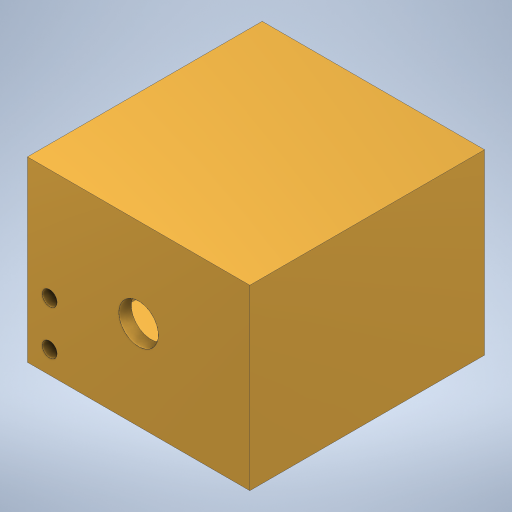
# Autodesk Inventor part: HUDISN-1-53
Saved by Autodesk Inventor 2024.2 (Build 282272000, 272)
## iProperties
Created: 2024-10-24
Part Number: HUDISN-1-53
Material: Generic
Document SubType Name: Modeling
Designer: Precisión-05
Density: 1 g/cm^3
Appearance: Default
Author: Precisión-05
Autodesk Inventor part; units mm, degrees
ref_plane "YZ Plane" through (0, 0, 0) normal (1, 0, 0) x (0, 1, 0)
ref_plane "XZ Plane" through (0, 0, 0) normal (0, 1, 0) x (-1, 0, 0)
ref_plane "XY Plane" through (0, 0, 0) normal (0, 0, 1) x (1, 0, 0)
sketch "Sketch1" plane through (0, 0, 0) normal (0, 1, 0) x (-1, 0, 0)
  line L0 (-22.5, 18) -> (22.5, 18)
  line L1 (22.5, 18) -> (22.5, -18)
  line L2 (22.5, -18) -> (-22.5, -18)
  line L3 (-22.5, -18) -> (-22.5, 18)
  line L4 (-22.5, 18) -> (22.5, -18) construction
  line L5 (22.5, 18) -> (-22.5, -18) construction
  line L6 (-22, 17.5) -> (22, 17.5)
  line L7 (22, 17.5) -> (22, -17.5)
  line L8 (22, -17.5) -> (-22, -17.5)
  line L9 (-22, -17.5) -> (-22, 17.5)
  line L10 (-22, 17.5) -> (22, -17.5) construction
  line L11 (22, 17.5) -> (-22, -17.5) construction
  point P0 (0, 0)
  dimension "d0" = 45
  dimension "d1" = 36
  dimension "d2" = 44
  dimension "d3" = 35
  constraints: 24 end point, 4 midpoint, 4 parallel, 2 horizontal, 2 perpendicular
  measures "d0" distance of L1.end L2.end
  measures "d1" distance of L0.end L1.end
  measures "d2" distance of L7.end L8.end
  measures "d3" distance of L6.end L7.end
extrude "Extrusion1" add sketch "Sketch1" along normal blind 2.5 contours L6 L7 L8 L9
extrude "Extrusion2" add sketch "Sketch1" along normal blind 47.5
sketch "Sketch2" plane through (0, 2.5, 0) normal (0, 1, 0) x (1, 0, 0)
  line L0 (-22.5, 18) -> (-22.5, -18) projected
  line L1 (22.5, 18) -> (-22.5, 18)
  line L2 (-22.5, 18) -> (-22.5, -18)
  line L3 (-22.5, -18) -> (22.5, -18)
  line L4 (22.5, -18) -> (22.5, 18)
  line L5 (22.5, 18) -> (-22.5, -18) construction
  line L6 (-22.5, 18) -> (22.5, -18) construction
  line L7 (22.5, 18) -> (-22.5, 18) projected
  line L8 (-22.5, 18) -> (-22.5, 13.5)
  line L9 (-22.5, 13.5) -> (-18, 13.5)
  line L10 (-18, 13.5) -> (-18, 4.5)
  point P0 (0, 0)
  point P1 (0, 0)
  dimension "d8" = 4.5
  dimension "d9" = 4.5
  dimension "d10" = 9
  constraints: 18 end point, 3 coincident, 3 perpendicular, 2 midpoint, 2 parallel, 1 horizontal, 1 point on line
  measures "d8" distance of L0.start L8.end
  measures "d9" distance of L8.end L9.end
  measures "d10" distance of L9.end L10.end
hole "Hole1" at (-18, 2.5, -4.5) at (-18, 2.5, -13.5) direction (0, -1, 0) diameter 3 depth 8
hole "Hole2" at (0, 2.5, 0) direction (0, -1, 0) diameter 8 depth 8
sketch "Sketch3" plane through (-22.5, 0, -18) normal (-1, 0, 0) x (0, 0, 1)
  line L0 (0, 0) -> (36, 0) projected
  line L1 (36, 0) -> (36, 47.5) projected
  line L2 (0, 47.5) -> (36, 47.5) projected
  line L3 (0, 0) -> (0, 47.5) projected
  line L4 (0, 47.5) -> (18, 47.5)
  line L5 (0, 47.5) -> (36, 47.5) projected
  line L6 (18, 47.5) -> (18, 39.5)
  line L7 (18, 39.5) -> (4, 39.5)
  line L8 (4, 39.5) -> (4, 33.5)
  point P0 (18, 0)
  dimension "d25" = 18
  dimension "d26" = 8
  dimension "d27" = 14
  dimension "d28" = 6
  constraints: 8 end point, 2 coincident, 2 perpendicular, 1 midpoint, 1 vertical
  measures "d25" distance of L2.start L4.end
  measures "d26" distance of L4.end L6.end
  measures "d27" distance of L6.end L7.end
  measures "d28" distance of L8.start L8.end
hole "Hole3" at (-22.5, 33.5, -14) at (-22.5, 39.5, -14) direction (1, 0, 0) diameter 2 depth 8
hole "Hole4" at (-22.5, 39.5, 0) direction (1, 0, 0) diameter 6 depth 8
thread "Thread1" size "M2x0.25" class "6H" standard "ANSI Metric M Profile" full length
thread "Thread2" size "M2x0.25" class "6H" standard "ANSI Metric M Profile" full length
body "Solid1"
